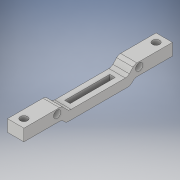
# Autodesk Inventor part: Frame_Mount
Saved by Autodesk Inventor 2019 (Build 230136000, 136)
## iProperties
Created: 2019-10-21
Part Number: Frame_Mount
Material: Generic
Document SubType Name: Modeling
Designer: 19879326
Density: 1 g/cm^3
Appearance: Default
Author: 19879326
Autodesk Inventor part; units mm, degrees
ref_plane "YZ Plane" through (0, 0, 0) normal (1, 0, 0) x (0, 1, 0)
ref_plane "XZ Plane" through (0, 0, 0) normal (0, 1, 0) x (-1, 0, 0)
ref_plane "XY Plane" through (0, 0, 0) normal (0, 0, 1) x (1, 0, 0)
sketch "Sketch1" plane through (0, 0, 0) normal (1, 0, 0) x (0, 1, 0)
  arc A0 (0, 49) -> (0, 41) centre (0, 45) ccw
  arc A1 (-1.4037, -41.2544) -> (-2.6656, -47.9824) centre (0, -45) ccw
  circle A2 centre (0, 45) radius 4
  circle A3 centre (0, -45) radius 4
  line L0 (5, 81.5) -> (-8, 81.5)
  line L1 (5, -81.5) -> (-8, -81.5)
  line L2 (5, -40) -> (-8, -40)
  line L3 (5, 40) -> (-8, 40)
  line L4 (5, 81.5) -> (5, 40)
  line L5 (5, -40) -> (5, -81.5)
  line L6 (-8, 81.5) -> (-8, 40)
  line L7 (-8, -40) -> (-8, -81.5)
  line L8 (-8, -40) -> (-13, -35.203)
  line L9 (-13, -35.203) -> (-13, 35.203)
  line L10 (-13, 35.203) -> (-8, 40)
  line L11 (5, 40) -> (-3, 32.3248)
  line L12 (-3, 32.3248) -> (-3, -32.3248)
  line L13 (-3, -32.3248) -> (5, -40)
  point P0 (0, 0)
  point P1 (0, 0)
  point P2 (-4, 45)
  point P3 (-8, -60.75)
  point P4 (-8, 60.75)
  point P5 (5, 60.75)
  dimension "d0" = 8
  dimension "d1" = 8
  dimension "d2" = 90
  dimension "d3" = 45
  dimension "d34" = 36.5
  dimension "d35" = 36.5
  dimension "d36" = 5
  dimension "d38" = 5
  dimension "d39" = 5
  dimension "d41" = 5
  dimension "d43" = 13
  dimension "d44" = 10
  dimension "d45" = 9
  dimension "d48" = 13
  constraints: 28 end point, 9 point on circle, 7 perpendicular, 4 centre point, 4 parallel, 3 coincident, 3 midpoint, 3 vertical alignment, 2 concentric, 1 equal length, 1 horizontal, 1 vertical
  measures "d0" diameter of A0
  measures "d1" diameter of A1
  measures "d2" distance of A1.centre A0.centre
  measures "d3" distance of point (0, 0) A1.centre
  measures "d34" distance from line of L1 A3.centre
  measures "d35" distance from line of L0 A2.centre
  measures "d36" distance from line of L2 A1.centre
  measures "d38" distance from line of A0.centre L3
  measures "d39" distance from line of point (0, 0) L5
  measures "d41" distance from line of L4 point (0, 0)
  measures "d43" distance of L1.start L1.end
  measures "d44" distance between parallel lines of L9 L12
  measures "d45" distance between parallel lines of L8 L13
  measures "d48" distance from line of L9 A1.centre
extrude "Extrusion1" add sketch "Sketch1" along normal blind 18
sketch "Sketch3" plane through (0, 5, 81.5) normal (0, 1, 0) x (1, 0, 0)
  circle A0 centre (9, 9) radius 4
  circle A1 centre (9, 154) radius 4
  line L0 (0, 41.5) -> (0, 0) projected
  line L1 (0, 0) -> (18, 0) projected
  line L2 (0, 163) -> (18, 163) projected
  point P0 (0, 81.5)
  dimension "d17" = 8
  dimension "d18" = 8
  dimension "d19" = 9
  dimension "d20" = 9
  dimension "d21" = 9
  constraints: 2 centre point, 1 vertical alignment
  measures "d17" diameter of A0
  measures "d18" diameter of A1
  measures "d19" distance from line of L0 A0.centre
  measures "d20" distance from line of L1 A0.centre
  measures "d21" distance from line of L2 A1.centre
extrude "Extrusion3" cut sketch "Sketch3" against normal blind 27.75
fillet "Fillet1" radius 6 8 edges at (9, -8, -40) (9, -13, -35.203) (9, -13, 35.203) (9, -8, 40) (9, 5, -40) (9, -3, -32.3248) (9, -3, 32.3248) (9, 5, 40)
sketch "Sketch5" plane through (0, -3, 29.7664) normal (0, 1, 0) x (1, 0, 0)
  line L0 (6, 54.5327) -> (12, 54.5327)
  line L1 (12, 54.5327) -> (12, 5)
  line L2 (12, 5) -> (6, 5)
  line L3 (6, 5) -> (6, 54.5327)
  line L4 (0, 111.2664) -> (18, 111.2664) projected
  line L5 (0, 59.5327) -> (18, 59.5327) projected
  line L6 (18, 0) -> (0, 0) projected
  point P0 (0, 29.7664)
  point P1 (9, 54.5327)
  point P2 (9, 111.2664)
  dimension "d49" = 6
  dimension "d50" = 5
  dimension "d51" = 5
  constraints: 8 end point, 2 midpoint, 2 parallel, 1 horizontal, 1 perpendicular, 1 vertical alignment
  measures "d49" distance of L0.start L0.end
  measures "d50" distance between parallel lines of L5 L0
  measures "d51" distance between parallel lines of L6 L2
extrude "Extrusion5" cut sketch "Sketch5" against normal blind 27.75
body "Solid1"
